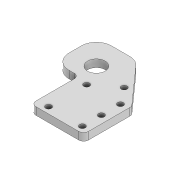
# Autodesk Inventor part: New_hinge_plate
Saved by Autodesk Inventor 2022 (Build 260153000, 153)
## iProperties
Created: 2022-07-14
Part Number: New_hinge_plate
Material: Generic
Document SubType Name: Modeling
Designer: dell
Density: 1 g/cm^3
Appearance: Default
Author: dell
Autodesk Inventor part; units mm, degrees
ref_plane "YZ Plane" through (0, 0, 0) normal (1, 0, 0) x (0, 1, 0)
ref_plane "XZ Plane" through (0, 0, 0) normal (0, 1, 0) x (-1, 0, 0)
ref_plane "XY Plane" through (0, 0, 0) normal (0, 0, 1) x (1, 0, 0)
sketch "Sketch1" plane through (0, 0, 0) normal (0, 1, 0) x (-1, 0, 0)
  line L0 (-10.5, 9.1) -> (10.5, 9.1)
  line L1 (10.5, 9.1) -> (10.5, -9.1)
  line L2 (10.5, -9.1) -> (-10.5, -9.1)
  line L3 (-10.5, -9.1) -> (-10.5, 9.1)
  line L4 (-10.5, 9.1) -> (10.5, -9.1) construction
  line L5 (10.5, 9.1) -> (-10.5, -9.1) construction
  line L6 (10.5, 9.1) -> (-10.5, 9.1)
  line L7 (-10.5, 9.1) -> (-10.5, 10.1)
  line L8 (-10.5, 10.1) -> (10.5, 10.1)
  line L9 (10.5, 10.1) -> (10.5, 9.1)
  line L10 (20.5, -26) -> (-10.5, -26)
  line L11 (-10.5, -26) -> (-10.5, -9.1)
  line L12 (-10.5, -9.1) -> (20.5, -9.1)
  line L13 (20.5, -9.1) -> (20.5, -26)
  circle A0 centre (10.5, -16) radius 3.5
  line L14 (-10.5, -9.1) -> (4.5, -26)
  circle A1 centre (6, -7.6) radius 1.15
  circle A2 centre (-7.5, -7.6) radius 1.15
  circle A3 centre (-7.5, 7.6) radius 1.15
  circle A4 centre (6, 7.6) radius 1.15
  circle A5 centre (-2.5, -14.1) radius 1.15
  circle A6 centre (-7.5, 0) radius 1.15
  point P0 (0, 0)
  point P1 (0, 0)
  point P2 (0, 0)
  point P3 (0, 0)
  dimension "d0" = 9.1
  dimension "d1" = 21
  dimension "d2" = 1
  dimension "d3" = 7
  dimension "d4" = 16
  dimension "d5" = 10
  dimension "d6" = 10
  dimension "d8" = 6
  dimension "d9" = 2.3
  dimension "d10" = 1.5
  dimension "d11" = 2.3
  dimension "d12" = 3
  dimension "d13" = 4.5
  dimension "d14" = 1.5
  dimension "d15" = 2.3
  dimension "d16" = 1.5
  dimension "d17" = 3
  dimension "d18" = 2.3
  dimension "d19" = 4.5
  dimension "d20" = 1.5
  dimension "d25" = 2.3
  dimension "d26" = 14.1
  dimension "d27" = 8
  dimension "d28" = 2.3
  dimension "d29" = 3
  constraints: 30 end point, 7 centre point, 6 parallel, 4 midpoint, 3 horizontal, 3 perpendicular, 3 point on line, 1 coincident, 1 collinear, 1 horizontal alignment
  measures "d0" distance from line of point (0, 0) L2
  measures "d1" distance between parallel lines of L3 L1
  measures "d2" distance between parallel lines of L0 L8
  measures "d3" diameter of A0
  measures "d4" vertical distance of point (0, 0) A0.centre
  measures "d5" distance from line of A0.centre L10
  measures "d6" distance from line of A0.centre L13
  measures "d8" horizontal distance of A0.centre L14.end
  measures "d9" diameter of A1
  measures "d10" distance from line of L2 A1.centre
  measures "d11" diameter of A2
  measures "d12" distance from line of L3 A2.centre
  measures "d13" distance from line of L1 A1.centre
  measures "d14" distance from line of L2 A2.centre
  measures "d15" diameter of A3
  measures "d16" distance from line of L6 A3.centre
  measures "d17" distance from line of L3 A3.centre
  measures "d18" diameter of A4
  measures "d19" distance from line of L1 A4.centre
  measures "d20" distance from line of L0 A4.centre
  measures "d25" diameter of A5
  measures "d26" vertical distance of point (0, 0) A5.centre
  measures "d27" distance from line of L3 A5.centre
  measures "d28" diameter of A6
  measures "d29" distance from line of L3 A6.centre
extrude "Extrusion1" add sketch "Sketch1" along normal blind 3 contours L7 L8 L9 L0 | L0 L1 L2 L3 | L2 L12 L13 L10 L14
fillet "Fillet1" radius 2 4 edges at (-10.5, 1.5, -9.1) (10.5, 1.5, -9.1) (10.5, 1.5, 10.1) (-10.5, 1.5, 10.1)
fillet "Fillet2" radius 6 3 edges at (-20.5, 1.5, -9.1) (-20.5, 1.5, -26) (-4.5, 1.5, -26)
body "Solid1"
